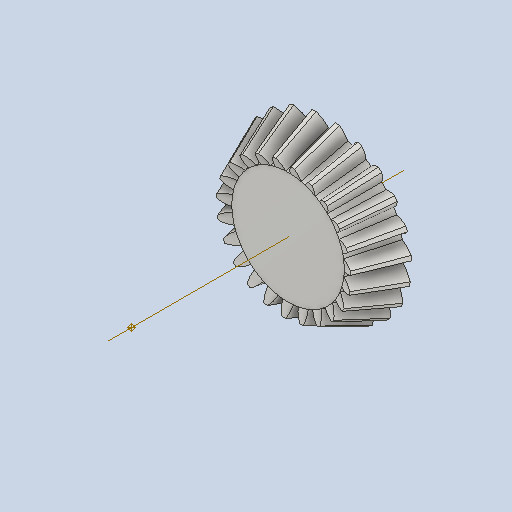
# Autodesk Inventor part: Bevel Gear1
Saved by Autodesk Inventor 2024 (Build 280153000, 153)
## iProperties
Created: 2024-04-16
Part Number: Bevel Gear1
Material: Steel, Mild
Document SubType Name: Modeling
Designer: teeta
Categories: <?xml version="1.0" encoding="UTF-16"?> <MemberInstance><Categories><FamilyTemplate><FamilyTemplateParameter ValueType="xs:double" Id="1" ObjectReferenceKey="da_z" ObjectType="kUserParameterObject"/><FamilyTemplateParameter ValueType="xs:double" Id="2" ObjectReferenceKey="da_b" ObjectType="kUserParameterObject"/><FamilyTemplateParameter ValueType="xs:double" Id="3" ObjectReferenceKey="da_beta" ObjectType="kUserParameterObject"/><FamilyTemplateParameter ValueType="xs:double" Id="4" ObjectReferenceKey="da_dae" ObjectType="kUserParameterObject"/><FamilyTemplateParameter ValueType="xs:double" Id="5" ObjectReferenceKey="da_ve" ObjectType="kUserParameterObject"/><FamilyTemplateParameter ValueType="xs:double" Id="6" ObjectReferenceKey="da_omega" ObjectType="kUserParameterObject"/><FamilyTemplateParameter ValueType="xs:string" Id="7" ObjectReferenceKey="EAIAABAAAAAAHwAAAAAAAIAAAAAAAAAA" ObjectType="83914240" SubObjectId="SurfaceGeometry"/></FamilyTemplate><ParamToTemplateMap><ParamToTemplate CategoryParameter="//CategoryParameter[@InternalName='046C89C9-8512-4d59-83FE-43B91F4F132A']" TemplateParameter="1"/><ParamToTemplate CategoryParameter="//CategoryParameter[@InternalName='2552DF32-E462-4b46-AEBF-C6C7768E72AC']" TemplateParameter="2"/><ParamToTemplate CategoryParameter="//CategoryParameter[@InternalName='C9EE641D-15FC-4fae-A226-E94C4372FDD7']" TemplateParameter="3"/><ParamToTemplate><ParamToTemplate CategoryParameter="//CategoryParameter[@InternalName='00B6519A-459B-49c7-AD84-2E56D39A5744']" ConstantValue="0.000000"/></ParamToTemplate><ParamToTemplate><ParamToTemplate CategoryParameter="//CategoryParameter[@InternalName='04B31F0E-C7A6-4894-AA32-9629BEFACF47']" ConstantValue="1.000000"/></ParamToTemplate><ParamToTemplate><ParamToTemplate CategoryParameter="//CategoryParameter[@InternalName='43CBEC2E-7847-49e7-A936-2F7889FCB2D9']" ConstantValue="0.200000"/></ParamToTemplate><ParamToTemplate><ParamToTemplate CategoryParameter="//CategoryParameter[@InternalName='B1EFC894-105D-4ebd-86BF-FA20ED196853']" ConstantValue="0.300000"/></ParamToTemplate><ParamToTemplate><ParamToTemplate CategoryParameter="//CategoryParameter[@InternalName='51175063-3D10-4879-93E8-6246FE8B403D']" ConstantValue="2060000000.000000"/></ParamToTemplate><ParamToTemplate><ParamToTemplate CategoryParameter="//CategoryParameter[@InternalName='A3A52E27-4454-46a9-B0BD-C932399B70AF']" ConstantValue="0.300000"/></ParamToTemplate><ParamToTemplate CategoryParameter="//CategoryParameter[@InternalName='2A200944-5A8C-41ca-B96E-8520D2E510F1']" TemplateParameter="4"/><ParamToTemplate><ParamToTemplate CategoryParameter="//CategoryParameter[@InternalName='1A637F62-92C8-44bc-B81F-10802510B579']" ConstantValue="5.838935"/></ParamToTemplate><ParamToTemplate CategoryParameter="//CategoryParameter[@InternalName='B52DD4BE-6863-48fb-BF58-89EF6F9EC65C']" TemplateParameter="5"/><ParamToTemplate><ParamToTemplate CategoryParameter="//CategoryParameter[@InternalName='3956BFF2-84D2-457d-93C2-9B0613DEBA67']" ConstantValue="6.607392"/></ParamToTemplate><ParamToTemplate CategoryParameter="//CategoryParameter[@InternalName='739CFA02-461B-4bf8-8049-181FCAD8B28F']" TemplateParameter="6"/><ParamToTemplate><ParamToTemplate CategoryParameter="//CategoryParameter[@InternalName='A27E999F-E2CE-4481-8A2A-EBF499C4C3C5']" ConstantValue="0.000000"/></ParamToTemplate><ParamToTemplate><ParamToTemplate CategoryParameter="//CategoryParameter[@InternalName='9E1B4470-B2D3-4ff1-B813-535BB4CDF51A']" ConstantValue="3520000.000000"/></ParamToTemplate><ParamToTemplate><ParamToTemplate CategoryParameter="//CategoryParameter[@InternalName='F8452263-BFF6-458c-9FB1-07C4B99E95CD']" ConstantValue="11400000.000000"/></ParamToTemplate><ParamToTemplate><ParamToTemplate CategoryParameter="//CategoryParameter[@InternalName='3E3BB259-FD49-497f-8171-6EBC954A3479']" ConstantValue="2.000000"/></ParamToTemplate><ParamToTemplate CategoryParameter="//CategoryParameter[@InternalName='27C3BAF2-7550-4e4b-AE2C-0DB134B7D9B7']" TemplateParameter="7"/></ParamToTemplateMap><Category DisplayName="Gear" InternalName="DC85795E-93AB-48d5-8EEE-5A27447B64BD" Mnemonic="Gear"><CategoryParameter DisplayName="z" InternalName="046C89C9-8512-4d59-83FE-43B91F4F132A" Mnemonic="z"/><CategoryParameter DisplayName="b" InternalName="2552DF32-E462-4b46-AEBF-C6C7768E72AC" Mnemonic="b"/><CategoryParameter DisplayName="||b|" InternalName="C9EE641D-15FC-4fae-A226-E94C4372FDD7" Mnemonic="beta"/><CategoryParameter DisplayName="x" InternalName="00B6519A-459B-49c7-AD84-2E56D39A5744" Mnemonic="x"/><CategoryParameter DisplayName="a*" InternalName="04B31F0E-C7A6-4894-AA32-9629BEFACF47" Mnemonic="a"/><CategoryParameter DisplayName="c*" InternalName="43CBEC2E-7847-49e7-A936-2F7889FCB2D9" Mnemonic="c"/><CategoryParameter DisplayName="r|.f|*" InternalName="B1EFC894-105D-4ebd-86BF-FA20ED196853" Mnemonic="rf"/><CategoryParameter DisplayName="E" InternalName="51175063-3D10-4879-93E8-6246FE8B403D" Mnemonic="E"/><CategoryParameter DisplayName="||m|" InternalName="A3A52E27-4454-46a9-B0BD-C932399B70AF" Mnemonic="mi"/><Category DisplayName="BevelGear" InternalName="0C98F69A-0C2B-4791-B2FE-7691BB227E77" Mnemonic="BevelGear"><CategoryParameter DisplayName="d|.ae|" InternalName="2A200944-5A8C-41ca-B96E-8520D2E510F1" Mnemonic="dae"/><CategoryParameter DisplayName="d|.ai|" InternalName="1A637F62-92C8-44bc-B81F-10802510B579" Mnemonic="dai"/><CategoryParameter DisplayName="A|.e|" InternalName="B52DD4BE-6863-48fb-BF58-89EF6F9EC65C" Mnemonic="ve"/><CategoryParameter DisplayName="A|.i|" InternalName="3956BFF2-84D2-457d-93C2-9B0613DEBA67" Mnemonic="vi"/><CategoryParameter DisplayName="||S|" InternalName="739CFA02-461B-4bf8-8049-181FCAD8B28F" Mnemonic="omega"/><CategoryParameter DisplayName="x|.t|" InternalName="A27E999F-E2CE-4481-8A2A-EBF499C4C3C5" Mnemonic="xt"/><CategoryParameter DisplayName="||s||.Flim|" InternalName="9E1B4470-B2D3-4ff1-B813-535BB4CDF51A" Mnemonic="sFlim"/><CategoryParameter DisplayName="||s||.Hlim|" InternalName="F8452263-BFF6-458c-9FB1-07C4B99E95CD" Mnemonic="sHlim"/><CategoryParameter DisplayName="type" InternalName="3E3BB259-FD49-497f-8171-6EBC954A3479" Mnemonic="type"/><CategoryParameter DisplayName="PitchDiameter" InternalName="27C3BAF2-7550-4e4b-AE2C-0DB134B7D9B7" Mnemonic="IDS_PITCHDIAM"/></Category></Category></Categories></MemberInstance>
Mass: 60.9118 g
Surface Area: 34.3074 cm^2
Volume: 7.7496 cm^3
Density: 7.86 g/cm^3
Appearance: Steel
CustomPartVersion: 1
Author: teeta
Autodesk Inventor part; units mm, degrees
ref_plane "Mesh Plane2" through (0, 0, 0) normal (0.9906859, 0.1361666, 0) x (0, 0, 1)
sketch "Teeth Body Sketch" plane through (0, 0, 0) normal (1, 0, 0) x (0, 1, 0)
  line L0 (0, 0) -> (31.161538, -86.847099) construction
  line L1 (31.161538, -86.847099) -> (37.282051, -84.377418)
  line L2 (37.282051, -84.377418) -> (0, 0) construction
  line L3 (34.5, -85.5) -> (0, 0) construction
  line L4 (24.40185, -68.007872) -> (29.194677, -66.073924)
  line L5 (31.161538, -86.847099) -> (24.40185, -68.007872)
  line L6 (37.282051, -84.377418) -> (29.194677, -66.073924)
  line L7 (0, -39.386751) -> (0, 6.564458)
  line L8 (0, -85.5) -> (37.282051, -85.5) construction
  dimension "d0" = 69
  dimension "d1" = 62.32308
  dimension "d2" = 74.5641
  dimension "d3" = 20
  dimension "d4" = 84.37742
  constraints: 16 end point, 4 point on line, 3 perpendicular, 2 collinear, 1 horizontal alignment, 1 vertical alignment
  measures "d0" diameter of L3.start L7
  measures "d1" diameter of L0.end L7
  measures "d2" diameter of L1.end L7
  measures "d3" distance between parallel lines of L1 L4
  measures "d4" vertical distance of L1.end L0.start
revolve "Teeth Body" add sketch "Teeth Body Sketch" angle 360 about axis through (0, 0, 0) along (0, 0, 1)
ref_plane "Tooth Plane" through (0, 34.5, -85.5) normal (0, -0.374194, 0.9273504) x (1, 0, 0)
sketch "Start Sketch" plane through (0, 34.5, -85.5) normal (0, -0.374194, 0.9273504) x (1, 0, 0)
  line L0 (0, -23.505131) -> (0, 10.644758)
  arc A0 (-1.242083, -4.391999) -> (-5.795531, 4.579977) centre (-14.921461, -5.693074) ccw
  arc A1 (5.795531, 4.579977) -> (1.242083, -4.391999) centre (14.921461, -5.693074) ccw
  line L1 (-1.242083, -4.391999) -> (1.242083, -4.391999)
  arc A2 (5.795531, 4.579977) -> (-5.795531, 4.579977) centre (0, -37.202764) ccw
  dimension "d7" = 13.74111
  dimension "d8" = 14.92146
  dimension "d9" = 31.50969
  dimension "d57" = 42.18276
  dimension "d58" = 32.81076
  constraints: 6 point on circle, 3 centre point, 3 symmetric about line, 2 end point, 1 coincident, 1 perpendicular, 1 other
  measures "d7" radius of A0
  measures "d8" horizontal distance of point (0, -37.203) A0.centre
  measures "d9" vertical distance of point (0, -37.203) A0.centre
  measures "d57" radius of A2
  measures "d58" distance from line of A2.centre L1
sketch "End Sketch" plane through (0, 26.892635, -66.646966) normal (0, -0.374194, 0.9273504) x (1, 0, 0)
  line L0 (0, -15.35404) -> (0, 6.953444)
  arc A0 (-0.968199, -3.423549) -> (-4.517597, 3.570076) centre (-11.631229, -4.437733) ccw
  arc A1 (4.517597, 3.570076) -> (0.968199, -3.423549) centre (11.631229, -4.437733) ccw
  line L1 (-0.968199, -3.423549) -> (0.968199, -3.423549)
  arc A2 (4.517597, 3.570076) -> (-4.517597, 3.570076) centre (0, -28.999431) ccw
  dimension "d12" = 10.71115
  dimension "d15" = 11.63123
  dimension "d16" = 24.5617
  dimension "d59" = 32.88132
  dimension "d60" = 25.57588
  constraints: 6 point on circle, 3 centre point, 3 symmetric about line, 2 end point, 1 coincident, 1 other
  measures "d12" radius of A0
  measures "d15" horizontal distance of A0.centre point (0, -28.999)
  measures "d16" vertical distance of A0.centre point (0, -28.999)
  measures "d59" radius of A2
  measures "d60" distance from line of A2.centre L1
loft "Loft" cut profiles "Start Sketch", "End Sketch"
pattern_circular "Circular Pattern" count 23 over 360 about axis through (0, 0, 0) along (0, 0, 1) of "Loft"
ref_plane "End Plane" through (0, 26.892635, -66.646966) normal (0, -0.374194, 0.9273504) x (1, 0, 0)
sketch3d "3D Sketch Right"
ref_plane "End Plane Right" through (-6.40738, 26.11818, -66.646966) normal (0.0891546, -0.363418, 0.9273504) x (0.971202, 0.2382578, 0)
sketch "End Sketch Right" plane through (-6.40738, 26.11818, -66.646966) normal (0.0891546, -0.363418, 0.9273504) x (0.971202, 0.2382578, 0)
  arc A0 (-0.968199, -3.423549) -> (-4.517597, 3.570076) centre (-11.631229, -4.437733) ccw
  line L0 (0, -39.511295) -> (0, 14.278518)
  arc A1 (4.517597, 3.570076) -> (0.968199, -3.423549) centre (11.631229, -4.437733) ccw
  line L1 (-0.968199, -3.423549) -> (0.968199, -3.423549)
  arc A2 (4.517597, 3.570076) -> (-4.517597, 3.570076) centre (0, -28.999431) ccw
  dimension "d70" = 11.63123
  dimension "d71" = 24.5617
  dimension "d72" = 10.71115
  dimension "d73" = 25.57588
  dimension "d74" = 32.88132
  constraints: 6 point on circle, 3 centre point, 3 symmetric about line, 2 end point, 1 coincident, 1 perpendicular, 1 other
  measures "d70" horizontal distance of A2.centre A0.centre
  measures "d71" vertical distance of point (0, -28.999) A0.centre
  measures "d72" radius of A0
  measures "d73" distance from line of point (0, -28.999) L1
  measures "d74" radius of A2
feature "Loft Right" [suppressed]
pattern_circular "Circular Pattern Right" [suppressed]
sketch3d "3D Sketch Left"
ref_plane "End Plane Left" through (6.388916, 26.11818, -66.640701) normal (-0.088907, -0.3634557, 0.9273594) x (0.9713606, -0.23761, 0)
sketch "End Sketch Left" plane through (6.388916, 26.11818, -66.640701) normal (-0.088907, -0.3634557, 0.9273594) x (0.9713606, -0.23761, 0)
  line L0 (0, -43.431417) -> (0, 18.202676)
  arc A0 (-0.968199, -3.42182) -> (-4.517597, 3.571806) centre (-11.631229, -4.436003) ccw
  arc A1 (4.517597, 3.571806) -> (0.968199, -3.42182) centre (11.631229, -4.436003) ccw
  line L1 (-0.968199, -3.42182) -> (0.968199, -3.42182)
  ellipse E0 centre (0, -24.722993) end of major axis (29.194677, -24.722993) minor radius 27.073959
  arc A2 (4.517597, 3.571806) -> (-4.517597, 3.571806) centre (0, -28.997702) ccw
  dimension "d56" = 27.07396
  dimension "d30" = 10.71115
  dimension "d31" = 11.63123
  dimension "d32" = 24.5617
  dimension "d61" = 32.88132
  dimension "d62" = 25.57588
  constraints: 6 point on circle, 3 centre point, 3 symmetric about line, 2 end point, 1 coincident, 2 other
  measures "d30" radius of A0
  measures "d31" horizontal distance of point (0, -28.998) A0.centre
  measures "d32" vertical distance of A0.centre point (0, -28.998)
  measures "d61" radius of A2
  measures "d62" distance from line of point (0, -28.998) L1
feature "Loft Left" [suppressed]
pattern_circular "Circular Pattern Left" [suppressed]
sketch "Body Sketch" plane through (0, 0, 0) normal (1, 0, 0) x (0, 1, 0)
  line L0 (0, -35.037536) -> (0, -19.530831)
  line L1 (31.161538, -86.847099) -> (24.40185, -68.007872)
  line L2 (24.40185, -68.007872) -> (0, -68.007872)
  line L3 (31.161538, -86.847099) -> (0, -86.847099)
  constraints: 4 end point, 2 perpendicular, 2 point on line
sketch "Body Sketch outline for Fix Body" plane through (0, 0, 0) normal (1, 0, 0) x (0, 1, 0)
  line L0 (0, -86.847099) -> (31.161538, -86.847099)
  line L1 (0, -68.007872) -> (0, -86.847099)
  line L2 (24.40185, -68.007872) -> (0, -68.007872)
  line L3 (31.161538, -86.847099) -> (24.40185, -68.007872)
revolve "Fix Body" add sketch "Body Sketch outline for Fix Body" angle 360 about axis through (0, 0, 0) along (0, 0, 1)
sketch "Sketch6" plane through (0, 0, 0) normal (1, 0, 0) x (0, 1, 0)
  line L0 (34.5, -85.5) -> (0, 0)
  line L1 (0, -37.799919) -> (0, 6.299986)
surface revolve "Pitch Diameter" sketch "Sketch6" angle 360 about axis through (0, 0, 0) along (0, 0, 1) shown no curves L0
equation "\"d0\" = da_de"
equation "\"d1\" = da_dfe"
equation "\"d2\" = da_dae"
equation "\"d3\" = da_b"
equation "\"d4\" = da_ve"
equation "\"d7\" = fd_rr"
equation "\"d8\" = fd_x"
equation "\"d9\" = fd_y"
equation "\"d57\" = 0.5 * fd_dva + 0.3 * da_he"
equation "\"d58\" = 0.5 * fd_dva - 1.12 * da_he"
equation "\"da_teethtype\" = 0"
equation "\"da_b\" = 20"
equation "\"da_de\" = 69"
equation "\"da_dae\" = 74.5641"
equation "\"da_dfe\" = 62.32308"
equation "\"da_le\" = 92.19816"
equation "\"da_omega\" = 90deg"
equation "\"da_beta\" = 0"
equation "\"da_delta\" = 21.974508deg"
equation "\"da_alpha\" = 20deg"
equation "\"da_he\" = 6.6"
equation "\"da_ve\" = 84.37742"
equation "\"da_zv\" = 24.801843"
equation "\"fd_loft\" = da_b + 0.05 * da_he"
equation "\"fd_x\" = fd_x1 + fd_x2"
equation "\"fd_y\" = fd_y1 - fd_y2"
equation "\"fd_dd\" = fd_dva - 0.8 * da_he"
equation "\"da_dvw\" = 74.40553"
equation "\"d11\" = fd_loft"
equation "\"da_dm\" = 61.51612"
equation "\"da_x\" = 0"
equation "\"da_m\" = 3"
equation "\"d50\" = da_omega"
equation "\"fd_rr\" = 13.741113"
equation "\"fd_dva\" = 80.40553"
equation "\"fd_x1\" = 2.380746"
equation "\"fd_x2\" = 12.540714"
equation "\"fd_y1\" = 37.12651"
equation "\"fd_y2\" = 5.61682"
body "Solid1"
body "Srf1"
